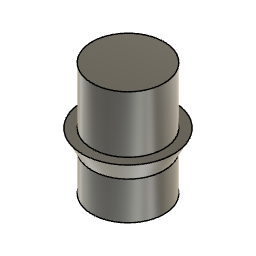
Final_CAD_Assembly (Autodesk Fusion 360 archive; units mm, degrees)
design "Button"
Autodesk Fusion 360 part; units mm, degrees
(part 1 of 3)
sketch "Sketch1" plane through (0, 0, 0) normal (0, 1, 0) x (1, 0, 0)
  line L0 (0, 0) -> (3.8, 0)
  line L1 (3.8, 0) -> (3.8, -12)
  line L2 (3.8, -12) -> (0, -12)
  line L3 (0, -12) -> (0, 0)
  line L4 (3.8, -6) -> (4.8, -6)
  line L5 (4.8, -6) -> (3.8, -4)
  line L6 (0, -0.5823) -> (0, -13.8484) construction
  dimension "d1" = 3.8
  dimension "d2" = 12
  dimension "d3" = 6
  dimension "d4" = 1
  dimension "d5" = 4
  constraint horizontal L0
  constraint vertical L1
  constraint horizontal L2
  constraint vertical L3
  constraint coincident L0.start L3.end
  constraint coincident L1 L4.start
  constraint perpendicular L1 L4
  constraint coincident L1 L5.end
  constraint coincident L3 L6.start
  constraint perpendicular L0 L6
  measures "d1" distance of L0.start L0.end
  measures "d2" distance of L0.start L2.end
  measures "d3" distance of L0 L4
  measures "d4" distance of L4.start L4.end
  measures "d5" distance of L0 L5.end
revolve "Revolve1" add sketch "Sketch1" angle 360 about axis through (0, 0, 0.5823) along (0, 0, 1)

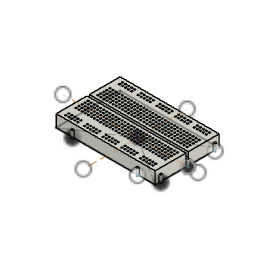
design "Breadboard"
Autodesk Fusion 360 part; units mm, degrees
sketch "Sketch1" plane through (0, 0, 0) normal (0, 0, 1) x (1, 0, 0)
  line L0 (41, 26.5) -> (-41, 26.5)
  line L1 (-41, 26.5) -> (-41, -26.5)
  line L2 (-41, -26.5) -> (41, -26.5)
  line L3 (41, -26.5) -> (41, 26.5)
  line L4 (41, 26.5) -> (-41, -26.5) construction
  line L5 (-41, 26.5) -> (41, -26.5) construction
  circle A0 centre (-27, -27.1) radius 1
  line L6 (0, 41) -> (0, -45) construction
  line L7 (50, 0) -> (-62, 0) construction
  circle A1 centre (27, -27.1) radius 1
  circle A2 centre (41.6, 0) radius 1
  circle A3 centre (41.6, -22.5) radius 1
  circle A4 centre (41.6, 22.5) radius 1
  dimension "d1" = 82
  dimension "d2" = 53
  dimension "d43" = 14
  dimension "d44" = 0.6
  dimension "d45" = 2
  dimension "d46" = 2
  dimension "d47" = 0.6
  dimension "d48" = 2
  dimension "d49" = 0.6
  dimension "d50" = 4
  constraint horizontal L0
  constraint perpendicular L0 L1
  constraint parallel L0 L2
  constraint parallel L1 L3
  constraint coincident L4 origin
  constraint coincident L5 origin
  constraint perpendicular L0 L6
  constraint perpendicular L3 L7
  constraint symmetric A0 L6 A1
  constraint coincident L7 A2.centre
  constraint symmetric L7 A3 A4
  measures "d1" distance of L0.start L0.end
  measures "d2" distance of L0.end L1.end
  measures "d43" distance of L1 A0.centre
  measures "d44" distance of L2 A0.centre
  measures "d45" diameter of A0
  measures "d46" diameter of A2
  measures "d47" distance of L3 A2.centre
  measures "d48" diameter of A3
  measures "d49" distance of L3 A3.centre
  measures "d50" distance of L2 A3.centre
extrude "Extrude1" add sketch "Sketch1" along normal blind 10 contours L0 L1 L2 L3 A0 A1 A2 A3 A4 | L3 A4 | L2 A0 | L3 A2 | L2 A1 | L3 A3 picked at (40.7957, 22.4762) picked at (-27.2307, -26.3971) picked at (40.7619, 0.2211) picked at (26.7693, -26.3971) picked at (40.7403, -22.5708)
sketch "Sketch2" plane through (0, 0, 10) normal (0, 0, 1) x (-1, 0, 0)
  line L0 (-41, 26.5) -> (-41, -26.5)
  line L1 (-41, -26.5) -> (41, -26.5)
  line L2 (41, -26.5) -> (41, 26.5)
  line L3 (41, 26.5) -> (-41, 26.5)
  line L4 (-41, -1) -> (41, -1)
  line L5 (41, -1) -> (41, 1)
  line L6 (41, 1) -> (-41, 1)
  line L7 (-41, 1) -> (-41, -1)
  line L8 (-41, -1) -> (41, 1) construction
  line L9 (41, -1) -> (-41, 1) construction
  line L10 (35.5, 23) -> (36.5, 23)
  line L11 (36.5, 23) -> (36.5, 24)
  line L12 (36.5, 24) -> (35.5, 24)
  line L13 (35.5, 24) -> (35.5, 23)
  line L14 (35.5, 23) -> (36.5, 24) construction
  line L15 (36.5, 23) -> (35.5, 24) construction
  line L16 (33, 24) -> (33, 23)
  line L17 (33, 23) -> (34, 23)
  line L18 (34, 23) -> (34, 24)
  line L19 (34, 24) -> (33, 24)
  line L20 (30.5, 24) -> (30.5, 23)
  line L21 (30.5, 23) -> (31.5, 23)
  line L22 (31.5, 23) -> (31.5, 24)
  line L23 (31.5, 24) -> (30.5, 24)
  line L24 (28, 24) -> (28, 23)
  line L25 (28, 23) -> (29, 23)
  line L26 (29, 23) -> (29, 24)
  line L27 (29, 24) -> (28, 24)
  line L28 (25.5, 24) -> (25.5, 23)
  line L29 (25.5, 23) -> (26.5, 23)
  line L30 (26.5, 23) -> (26.5, 24)
  line L31 (26.5, 24) -> (25.5, 24)
  line L32 (35.5, 21.5) -> (35.5, 20.5)
  line L33 (35.5, 20.5) -> (36.5, 20.5)
  line L34 (36.5, 20.5) -> (36.5, 21.5)
  line L35 (36.5, 21.5) -> (35.5, 21.5)
  line L36 (33, 21.5) -> (33, 20.5)
  line L37 (33, 20.5) -> (34, 20.5)
  line L38 (34, 20.5) -> (34, 21.5)
  line L39 (34, 21.5) -> (33, 21.5)
  line L40 (30.5, 21.5) -> (30.5, 20.5)
  line L41 (30.5, 20.5) -> (31.5, 20.5)
  line L42 (31.5, 20.5) -> (31.5, 21.5)
  line L43 (31.5, 21.5) -> (30.5, 21.5)
  line L44 (28, 21.5) -> (28, 20.5)
  line L45 (28, 20.5) -> (29, 20.5)
  line L46 (29, 20.5) -> (29, 21.5)
  line L47 (29, 21.5) -> (28, 21.5)
  line L48 (25.5, 21.5) -> (25.5, 20.5)
  line L49 (25.5, 20.5) -> (26.5, 20.5)
  line L50 (26.5, 20.5) -> (26.5, 21.5)
  line L51 (26.5, 21.5) -> (25.5, 21.5)
  line L52 (17.5, 23) -> (18.5, 23)
  line L53 (12.5, 24) -> (12.5, 23)
  line L54 (20, 23) -> (21, 23)
  line L55 (16, 21.5) -> (15, 21.5)
  line L56 (13.5, 23) -> (13.5, 24)
  line L57 (12.5, 21.5) -> (12.5, 20.5)
  line L58 (20, 23) -> (21, 24) construction
  line L59 (12.5, 23) -> (13.5, 23)
  line L60 (20, 20.5) -> (21, 20.5)
  line L61 (21, 24) -> (20, 24)
  line L62 (18.5, 23) -> (18.5, 24)
  line L63 (20, 24) -> (20, 23)
  line L64 (12.5, 20.5) -> (13.5, 20.5)
  line L65 (16, 23) -> (16, 24)
  line L66 (15, 23) -> (16, 23)
  line L67 (18.5, 20.5) -> (18.5, 21.5)
  line L68 (15, 21.5) -> (15, 20.5)
  line L69 (13.5, 24) -> (12.5, 24)
  line L70 (16, 24) -> (15, 24)
  line L71 (13.5, 21.5) -> (12.5, 21.5)
  line L72 (21, 21.5) -> (20, 21.5)
  line L73 (21, 20.5) -> (21, 21.5)
  line L74 (21, 23) -> (21, 24)
  line L75 (10, 21.5) -> (10, 20.5)
  line L76 (11, 23) -> (11, 24)
  line L77 (11, 24) -> (10, 24)
  line L78 (10, 24) -> (10, 23)
  line L79 (11, 21.5) -> (10, 21.5)
  line L80 (11, 20.5) -> (11, 21.5)
  line L81 (10, 23) -> (11, 23)
  line L82 (18.5, 24) -> (17.5, 24)
  line L83 (15, 20.5) -> (16, 20.5)
  line L84 (15, 24) -> (15, 23)
  line L85 (20, 21.5) -> (20, 20.5)
  line L86 (17.5, 24) -> (17.5, 23)
  line L87 (17.5, 21.5) -> (17.5, 20.5)
  line L88 (21, 23) -> (20, 24) construction
  line L89 (13.5, 20.5) -> (13.5, 21.5)
  line L90 (16, 20.5) -> (16, 21.5)
  line L91 (18.5, 21.5) -> (17.5, 21.5)
  line L92 (17.5, 20.5) -> (18.5, 20.5)
  line L93 (10, 20.5) -> (11, 20.5)
  line L94 (2, 23) -> (3, 23)
  line L95 (-3, 24) -> (-3, 23)
  line L96 (4.5, 23) -> (5.5, 23)
  line L97 (0.5, 21.5) -> (-0.5, 21.5)
  line L98 (-2, 23) -> (-2, 24)
  line L99 (-3, 21.5) -> (-3, 20.5)
  line L100 (4.5, 23) -> (5.5, 24) construction
  line L101 (-3, 23) -> (-2, 23)
  line L102 (4.5, 20.5) -> (5.5, 20.5)
  line L103 (5.5, 24) -> (4.5, 24)
  line L104 (3, 23) -> (3, 24)
  line L105 (4.5, 24) -> (4.5, 23)
  line L106 (-3, 20.5) -> (-2, 20.5)
  line L107 (0.5, 23) -> (0.5, 24)
  line L108 (-0.5, 23) -> (0.5, 23)
  line L109 (3, 20.5) -> (3, 21.5)
  line L110 (-0.5, 21.5) -> (-0.5, 20.5)
  line L111 (-2, 24) -> (-3, 24)
  line L112 (0.5, 24) -> (-0.5, 24)
  line L113 (-2, 21.5) -> (-3, 21.5)
  line L114 (5.5, 21.5) -> (4.5, 21.5)
  line L115 (5.5, 20.5) -> (5.5, 21.5)
  line L116 (5.5, 23) -> (5.5, 24)
  line L117 (-5.5, 21.5) -> (-5.5, 20.5)
  line L118 (-4.5, 23) -> (-4.5, 24)
  line L119 (-4.5, 24) -> (-5.5, 24)
  line L120 (-5.5, 24) -> (-5.5, 23)
  line L121 (-4.5, 21.5) -> (-5.5, 21.5)
  line L122 (-4.5, 20.5) -> (-4.5, 21.5)
  line L123 (-5.5, 23) -> (-4.5, 23)
  line L124 (3, 24) -> (2, 24)
  line L125 (-0.5, 20.5) -> (0.5, 20.5)
  line L126 (-0.5, 24) -> (-0.5, 23)
  line L127 (4.5, 21.5) -> (4.5, 20.5)
  line L128 (2, 24) -> (2, 23)
  line L129 (2, 21.5) -> (2, 20.5)
  line L130 (5.5, 23) -> (4.5, 24) construction
  line L131 (-2, 20.5) -> (-2, 21.5)
  line L132 (0.5, 20.5) -> (0.5, 21.5)
  line L133 (3, 21.5) -> (2, 21.5)
  line L134 (2, 20.5) -> (3, 20.5)
  line L135 (-5.5, 20.5) -> (-4.5, 20.5)
  line L136 (-13.5, 23) -> (-12.5, 23)
  line L137 (-18.5, 24) -> (-18.5, 23)
  line L138 (-11, 23) -> (-10, 23)
  line L139 (-15, 21.5) -> (-16, 21.5)
  line L140 (-17.5, 23) -> (-17.5, 24)
  line L141 (-18.5, 21.5) -> (-18.5, 20.5)
  line L142 (-11, 23) -> (-10, 24) construction
  line L143 (-18.5, 23) -> (-17.5, 23)
  line L144 (-11, 20.5) -> (-10, 20.5)
  line L145 (-10, 24) -> (-11, 24)
  line L146 (-12.5, 23) -> (-12.5, 24)
  line L147 (-11, 24) -> (-11, 23)
  line L148 (-18.5, 20.5) -> (-17.5, 20.5)
  line L149 (-15, 23) -> (-15, 24)
  line L150 (-16, 23) -> (-15, 23)
  line L151 (-12.5, 20.5) -> (-12.5, 21.5)
  line L152 (-16, 21.5) -> (-16, 20.5)
  line L153 (-17.5, 24) -> (-18.5, 24)
  line L154 (-15, 24) -> (-16, 24)
  line L155 (-17.5, 21.5) -> (-18.5, 21.5)
  line L156 (-10, 21.5) -> (-11, 21.5)
  line L157 (-10, 20.5) -> (-10, 21.5)
  line L158 (-10, 23) -> (-10, 24)
  line L159 (-21, 21.5) -> (-21, 20.5)
  line L160 (-20, 23) -> (-20, 24)
  line L161 (-20, 24) -> (-21, 24)
  line L162 (-21, 24) -> (-21, 23)
  line L163 (-20, 21.5) -> (-21, 21.5)
  line L164 (-20, 20.5) -> (-20, 21.5)
  line L165 (-21, 23) -> (-20, 23)
  line L166 (-12.5, 24) -> (-13.5, 24)
  line L167 (-16, 20.5) -> (-15, 20.5)
  line L168 (-16, 24) -> (-16, 23)
  line L169 (-11, 21.5) -> (-11, 20.5)
  line L170 (-13.5, 24) -> (-13.5, 23)
  line L171 (-13.5, 21.5) -> (-13.5, 20.5)
  line L172 (-10, 23) -> (-11, 24) construction
  line L173 (-17.5, 20.5) -> (-17.5, 21.5)
  line L174 (-15, 20.5) -> (-15, 21.5)
  line L175 (-12.5, 21.5) -> (-13.5, 21.5)
  line L176 (-13.5, 20.5) -> (-12.5, 20.5)
  line L177 (-21, 20.5) -> (-20, 20.5)
  line L178 (-29, 23) -> (-28, 23)
  line L179 (-34, 24) -> (-34, 23)
  line L180 (-26.5, 23) -> (-25.5, 23)
  line L181 (-30.5, 21.5) -> (-31.5, 21.5)
  line L182 (-33, 23) -> (-33, 24)
  line L183 (-34, 21.5) -> (-34, 20.5)
  line L184 (-26.5, 23) -> (-25.5, 24) construction
  line L185 (-34, 23) -> (-33, 23)
  line L186 (-26.5, 20.5) -> (-25.5, 20.5)
  line L187 (-25.5, 24) -> (-26.5, 24)
  line L188 (-28, 23) -> (-28, 24)
  line L189 (-26.5, 24) -> (-26.5, 23)
  line L190 (-34, 20.5) -> (-33, 20.5)
  line L191 (-30.5, 23) -> (-30.5, 24)
  line L192 (-31.5, 23) -> (-30.5, 23)
  line L193 (-28, 20.5) -> (-28, 21.5)
  line L194 (-31.5, 21.5) -> (-31.5, 20.5)
  line L195 (-33, 24) -> (-34, 24)
  line L196 (-30.5, 24) -> (-31.5, 24)
  line L197 (-33, 21.5) -> (-34, 21.5)
  line L198 (-25.5, 21.5) -> (-26.5, 21.5)
  line L199 (-25.5, 20.5) -> (-25.5, 21.5)
  line L200 (-25.5, 23) -> (-25.5, 24)
  line L201 (-36.5, 21.5) -> (-36.5, 20.5)
  line L202 (-35.5, 23) -> (-35.5, 24)
  line L203 (-35.5, 24) -> (-36.5, 24)
  line L204 (-36.5, 24) -> (-36.5, 23)
  line L205 (-35.5, 21.5) -> (-36.5, 21.5)
  line L206 (-35.5, 20.5) -> (-35.5, 21.5)
  line L207 (-36.5, 23) -> (-35.5, 23)
  line L208 (-28, 24) -> (-29, 24)
  line L209 (-31.5, 20.5) -> (-30.5, 20.5)
  line L210 (-31.5, 24) -> (-31.5, 23)
  line L211 (-26.5, 21.5) -> (-26.5, 20.5)
  line L212 (-29, 24) -> (-29, 23)
  line L213 (-29, 21.5) -> (-29, 20.5)
  line L214 (-25.5, 23) -> (-26.5, 24) construction
  line L215 (-33, 20.5) -> (-33, 21.5)
  line L216 (-30.5, 20.5) -> (-30.5, 21.5)
  line L217 (-28, 21.5) -> (-29, 21.5)
  line L218 (-29, 20.5) -> (-28, 20.5)
  line L219 (-36.5, 20.5) -> (-35.5, 20.5)
  line L220 (36.5, 4.5) -> (37.5, 4.5)
  line L221 (37.5, 4.5) -> (37.5, 3.5)
  line L222 (37.5, 3.5) -> (36.5, 3.5)
  line L223 (36.5, 3.5) -> (36.5, 4.5)
  line L224 (36.5, 4.5) -> (37.5, 3.5) construction
  line L225 (37.5, 4.5) -> (36.5, 3.5) construction
  line L226 (33.9483, 3.5) -> (33.9483, 4.5)
  line L227 (34.9483, 3.5) -> (33.9483, 3.5)
  line L228 (34.9483, 4.5) -> (34.9483, 3.5)
  line L229 (33.9483, 4.5) -> (34.9483, 4.5)
  line L230 (31.3966, 3.5) -> (31.3966, 4.5)
  line L231 (32.3966, 3.5) -> (31.3966, 3.5)
  line L232 (32.3966, 4.5) -> (32.3966, 3.5)
  line L233 (31.3966, 4.5) -> (32.3966, 4.5)
  line L234 (28.8448, 3.5) -> (28.8448, 4.5)
  line L235 (29.8448, 3.5) -> (28.8448, 3.5)
  line L236 (29.8448, 4.5) -> (29.8448, 3.5)
  line L237 (28.8448, 4.5) -> (29.8448, 4.5)
  line L238 (26.2931, 3.5) -> (26.2931, 4.5)
  line L239 (27.2931, 3.5) -> (26.2931, 3.5)
  line L240 (27.2931, 4.5) -> (27.2931, 3.5)
  line L241 (26.2931, 4.5) -> (27.2931, 4.5)
  line L242 (23.7414, 3.5) -> (23.7414, 4.5)
  line L243 (24.7414, 3.5) -> (23.7414, 3.5)
  line L244 (24.7414, 4.5) -> (24.7414, 3.5)
  line L245 (23.7414, 4.5) -> (24.7414, 4.5)
  line L246 (21.1897, 3.5) -> (21.1897, 4.5)
  line L247 (22.1897, 3.5) -> (21.1897, 3.5)
  line L248 (22.1897, 4.5) -> (22.1897, 3.5)
  line L249 (21.1897, 4.5) -> (22.1897, 4.5)
  line L250 (18.6379, 3.5) -> (18.6379, 4.5)
  line L251 (19.6379, 3.5) -> (18.6379, 3.5)
  line L252 (19.6379, 4.5) -> (19.6379, 3.5)
  line L253 (18.6379, 4.5) -> (19.6379, 4.5)
  line L254 (16.0862, 3.5) -> (16.0862, 4.5)
  line L255 (17.0862, 3.5) -> (16.0862, 3.5)
  line L256 (17.0862, 4.5) -> (17.0862, 3.5)
  line L257 (16.0862, 4.5) -> (17.0862, 4.5)
  line L258 (13.5345, 3.5) -> (13.5345, 4.5)
  line L259 (14.5345, 3.5) -> (13.5345, 3.5)
  line L260 (14.5345, 4.5) -> (14.5345, 3.5)
  line L261 (13.5345, 4.5) -> (14.5345, 4.5)
  line L262 (10.9828, 3.5) -> (10.9828, 4.5)
  line L263 (11.9828, 3.5) -> (10.9828, 3.5)
  line L264 (11.9828, 4.5) -> (11.9828, 3.5)
  line L265 (10.9828, 4.5) -> (11.9828, 4.5)
  line L266 (8.431, 3.5) -> (8.431, 4.5)
  line L267 (9.431, 3.5) -> (8.431, 3.5)
  line L268 (9.431, 4.5) -> (9.431, 3.5)
  line L269 (8.431, 4.5) -> (9.431, 4.5)
  line L270 (5.8793, 3.5) -> (5.8793, 4.5)
  line L271 (6.8793, 3.5) -> (5.8793, 3.5)
  line L272 (6.8793, 4.5) -> (6.8793, 3.5)
  line L273 (5.8793, 4.5) -> (6.8793, 4.5)
  line L274 (3.3276, 3.5) -> (3.3276, 4.5)
  line L275 (4.3276, 3.5) -> (3.3276, 3.5)
  line L276 (4.3276, 4.5) -> (4.3276, 3.5)
  line L277 (3.3276, 4.5) -> (4.3276, 4.5)
  line L278 (0.7759, 3.5) -> (0.7759, 4.5)
  line L279 (1.7759, 3.5) -> (0.7759, 3.5)
  line L280 (1.7759, 4.5) -> (1.7759, 3.5)
  line L281 (0.7759, 4.5) -> (1.7759, 4.5)
  line L282 (-1.7759, 3.5) -> (-1.7759, 4.5)
  line L283 (-0.7759, 3.5) -> (-1.7759, 3.5)
  line L284 (-0.7759, 4.5) -> (-0.7759, 3.5)
  line L285 (-1.7759, 4.5) -> (-0.7759, 4.5)
  line L286 (-4.3276, 3.5) -> (-4.3276, 4.5)
  line L287 (-3.3276, 3.5) -> (-4.3276, 3.5)
  line L288 (-3.3276, 4.5) -> (-3.3276, 3.5)
  line L289 (-4.3276, 4.5) -> (-3.3276, 4.5)
  line L290 (-6.8793, 3.5) -> (-6.8793, 4.5)
  line L291 (-5.8793, 3.5) -> (-6.8793, 3.5)
  line L292 (-5.8793, 4.5) -> (-5.8793, 3.5)
  line L293 (-6.8793, 4.5) -> (-5.8793, 4.5)
  line L294 (-9.431, 3.5) -> (-9.431, 4.5)
  line L295 (-8.431, 3.5) -> (-9.431, 3.5)
  line L296 (-8.431, 4.5) -> (-8.431, 3.5)
  line L297 (-9.431, 4.5) -> (-8.431, 4.5)
  line L298 (-11.9828, 3.5) -> (-11.9828, 4.5)
  line L299 (-10.9828, 3.5) -> (-11.9828, 3.5)
  line L300 (-10.9828, 4.5) -> (-10.9828, 3.5)
  line L301 (-11.9828, 4.5) -> (-10.9828, 4.5)
  line L302 (-14.5345, 3.5) -> (-14.5345, 4.5)
  line L303 (-13.5345, 3.5) -> (-14.5345, 3.5)
  line L304 (-13.5345, 4.5) -> (-13.5345, 3.5)
  line L305 (-14.5345, 4.5) -> (-13.5345, 4.5)
  line L306 (-17.0862, 3.5) -> (-17.0862, 4.5)
  line L307 (-16.0862, 3.5) -> (-17.0862, 3.5)
  line L308 (-16.0862, 4.5) -> (-16.0862, 3.5)
  line L309 (-17.0862, 4.5) -> (-16.0862, 4.5)
  line L310 (-19.6379, 3.5) -> (-19.6379, 4.5)
  line L311 (-18.6379, 3.5) -> (-19.6379, 3.5)
  line L312 (-18.6379, 4.5) -> (-18.6379, 3.5)
  line L313 (-19.6379, 4.5) -> (-18.6379, 4.5)
  line L314 (-22.1897, 3.5) -> (-22.1897, 4.5)
  line L315 (-21.1897, 3.5) -> (-22.1897, 3.5)
  line L316 (-21.1897, 4.5) -> (-21.1897, 3.5)
  line L317 (-22.1897, 4.5) -> (-21.1897, 4.5)
  line L318 (-24.7414, 3.5) -> (-24.7414, 4.5)
  line L319 (-23.7414, 3.5) -> (-24.7414, 3.5)
  line L320 (-23.7414, 4.5) -> (-23.7414, 3.5)
  line L321 (-24.7414, 4.5) -> (-23.7414, 4.5)
  line L322 (-27.2931, 3.5) -> (-27.2931, 4.5)
  line L323 (-26.2931, 3.5) -> (-27.2931, 3.5)
  line L324 (-26.2931, 4.5) -> (-26.2931, 3.5)
  line L325 (-27.2931, 4.5) -> (-26.2931, 4.5)
  line L326 (-29.8448, 3.5) -> (-29.8448, 4.5)
  line L327 (-28.8448, 3.5) -> (-29.8448, 3.5)
  line L328 (-28.8448, 4.5) -> (-28.8448, 3.5)
  line L329 (-29.8448, 4.5) -> (-28.8448, 4.5)
  line L330 (-32.3966, 3.5) -> (-32.3966, 4.5)
  line L331 (-31.3966, 3.5) -> (-32.3966, 3.5)
  line L332 (-31.3966, 4.5) -> (-31.3966, 3.5)
  line L333 (-32.3966, 4.5) -> (-31.3966, 4.5)
  line L334 (-34.9483, 3.5) -> (-34.9483, 4.5)
  line L335 (-33.9483, 3.5) -> (-34.9483, 3.5)
  line L336 (-33.9483, 4.5) -> (-33.9483, 3.5)
  line L337 (-34.9483, 4.5) -> (-33.9483, 4.5)
  line L338 (-37.5, 3.5) -> (-37.5, 4.5)
  line L339 (-36.5, 3.5) -> (-37.5, 3.5)
  line L340 (-36.5, 4.5) -> (-36.5, 3.5)
  line L341 (-37.5, 4.5) -> (-36.5, 4.5)
  line L342 (36.5, 6) -> (36.5, 7)
  line L343 (37.5, 6) -> (36.5, 6)
  line L344 (37.5, 7) -> (37.5, 6)
  line L345 (36.5, 7) -> (37.5, 7)
  line L346 (33.9483, 6) -> (33.9483, 7)
  line L347 (34.9483, 6) -> (33.9483, 6)
  line L348 (34.9483, 7) -> (34.9483, 6)
  line L349 (33.9483, 7) -> (34.9483, 7)
  line L350 (31.3966, 6) -> (31.3966, 7)
  line L351 (32.3966, 6) -> (31.3966, 6)
  line L352 (32.3966, 7) -> (32.3966, 6)
  line L353 (31.3966, 7) -> (32.3966, 7)
  line L354 (28.8448, 6) -> (28.8448, 7)
  line L355 (29.8448, 6) -> (28.8448, 6)
  line L356 (29.8448, 7) -> (29.8448, 6)
  line L357 (28.8448, 7) -> (29.8448, 7)
  line L358 (26.2931, 6) -> (26.2931, 7)
  line L359 (27.2931, 6) -> (26.2931, 6)
  line L360 (27.2931, 7) -> (27.2931, 6)
  line L361 (26.2931, 7) -> (27.2931, 7)
  line L362 (23.7414, 6) -> (23.7414, 7)
  line L363 (24.7414, 6) -> (23.7414, 6)
  line L364 (24.7414, 7) -> (24.7414, 6)
  line L365 (23.7414, 7) -> (24.7414, 7)
  line L366 (21.1897, 6) -> (21.1897, 7)
  line L367 (22.1897, 6) -> (21.1897, 6)
  line L368 (22.1897, 7) -> (22.1897, 6)
  line L369 (21.1897, 7) -> (22.1897, 7)
  line L370 (18.6379, 6) -> (18.6379, 7)
  line L371 (19.6379, 6) -> (18.6379, 6)
  line L372 (19.6379, 7) -> (19.6379, 6)
  line L373 (18.6379, 7) -> (19.6379, 7)
  line L374 (16.0862, 6) -> (16.0862, 7)
  line L375 (17.0862, 6) -> (16.0862, 6)
  line L376 (17.0862, 7) -> (17.0862, 6)
  line L377 (16.0862, 7) -> (17.0862, 7)
  line L378 (13.5345, 6) -> (13.5345, 7)
  line L379 (14.5345, 6) -> (13.5345, 6)
  line L380 (14.5345, 7) -> (14.5345, 6)
  line L381 (13.5345, 7) -> (14.5345, 7)
  line L382 (10.9828, 6) -> (10.9828, 7)
  line L383 (11.9828, 6) -> (10.9828, 6)
  line L384 (11.9828, 7) -> (11.9828, 6)
  line L385 (10.9828, 7) -> (11.9828, 7)
  line L386 (8.431, 6) -> (8.431, 7)
  line L387 (9.431, 6) -> (8.431, 6)
  line L388 (9.431, 7) -> (9.431, 6)
  line L389 (8.431, 7) -> (9.431, 7)
  line L390 (5.8793, 6) -> (5.8793, 7)
  line L391 (6.8793, 6) -> (5.8793, 6)
  line L392 (6.8793, 7) -> (6.8793, 6)
  line L393 (5.8793, 7) -> (6.8793, 7)
  line L394 (3.3276, 6) -> (3.3276, 7)
  line L395 (4.3276, 6) -> (3.3276, 6)
  line L396 (4.3276, 7) -> (4.3276, 6)
  line L397 (3.3276, 7) -> (4.3276, 7)
  line L398 (0.7759, 6) -> (0.7759, 7)
  line L399 (1.7759, 6) -> (0.7759, 6)
  line L400 (1.7759, 7) -> (1.7759, 6)
  line L401 (0.7759, 7) -> (1.7759, 7)
  line L402 (-1.7759, 6) -> (-1.7759, 7)
  line L403 (-0.7759, 6) -> (-1.7759, 6)
  line L404 (-0.7759, 7) -> (-0.7759, 6)
  line L405 (-1.7759, 7) -> (-0.7759, 7)
  line L406 (-4.3276, 6) -> (-4.3276, 7)
  line L407 (-3.3276, 6) -> (-4.3276, 6)
  line L408 (-3.3276, 7) -> (-3.3276, 6)
  line L409 (-4.3276, 7) -> (-3.3276, 7)
  line L410 (-6.8793, 6) -> (-6.8793, 7)
  line L411 (-5.8793, 6) -> (-6.8793, 6)
  line L412 (-5.8793, 7) -> (-5.8793, 6)
  line L413 (-6.8793, 7) -> (-5.8793, 7)
  line L414 (-9.431, 6) -> (-9.431, 7)
  line L415 (-8.431, 6) -> (-9.431, 6)
  line L416 (-8.431, 7) -> (-8.431, 6)
  line L417 (-9.431, 7) -> (-8.431, 7)
  line L418 (-11.9828, 6) -> (-11.9828, 7)
  line L419 (-10.9828, 6) -> (-11.9828, 6)
  line L420 (-10.9828, 7) -> (-10.9828, 6)
  line L421 (-11.9828, 7) -> (-10.9828, 7)
  line L422 (-14.5345, 6) -> (-14.5345, 7)
  line L423 (-13.5345, 6) -> (-14.5345, 6)
  line L424 (-13.5345, 7) -> (-13.5345, 6)
  line L425 (-14.5345, 7) -> (-13.5345, 7)
  line L426 (-17.0862, 6) -> (-17.0862, 7)
  line L427 (-16.0862, 6) -> (-17.0862, 6)
  line L428 (-16.0862, 7) -> (-16.0862, 6)
  line L429 (-17.0862, 7) -> (-16.0862, 7)
  line L430 (-19.6379, 6) -> (-19.6379, 7)
  line L431 (-18.6379, 6) -> (-19.6379, 6)
  line L432 (-18.6379, 7) -> (-18.6379, 6)
  line L433 (-19.6379, 7) -> (-18.6379, 7)
  line L434 (-22.1897, 6) -> (-22.1897, 7)
  line L435 (-21.1897, 6) -> (-22.1897, 6)
  line L436 (-21.1897, 7) -> (-21.1897, 6)
  line L437 (-22.1897, 7) -> (-21.1897, 7)
  line L438 (-24.7414, 6) -> (-24.7414, 7)
  line L439 (-23.7414, 6) -> (-24.7414, 6)
  line L440 (-23.7414, 7) -> (-23.7414, 6)
  line L441 (-24.7414, 7) -> (-23.7414, 7)
  line L442 (-27.2931, 6) -> (-27.2931, 7)
  line L443 (-26.2931, 6) -> (-27.2931, 6)
  line L444 (-26.2931, 7) -> (-26.2931, 6)
  line L445 (-27.2931, 7) -> (-26.2931, 7)
  line L446 (-29.8448, 6) -> (-29.8448, 7)
  line L447 (-28.8448, 6) -> (-29.8448, 6)
  line L448 (-28.8448, 7) -> (-28.8448, 6)
  line L449 (-29.8448, 7) -> (-28.8448, 7)
  line L450 (-32.3966, 6) -> (-32.3966, 7)
  line L451 (-31.3966, 6) -> (-32.3966, 6)
  line L452 (-31.3966, 7) -> (-31.3966, 6)
  line L453 (-32.3966, 7) -> (-31.3966, 7)
  line L454 (-34.9483, 6) -> (-34.9483, 7)
  line L455 (-33.9483, 6) -> (-34.9483, 6)
  line L456 (-33.9483, 7) -> (-33.9483, 6)
  line L457 (-34.9483, 7) -> (-33.9483, 7)
  line L458 (-37.5, 6) -> (-37.5, 7)
  line L459 (-36.5, 6) -> (-37.5, 6)
  line L460 (-36.5, 7) -> (-36.5, 6)
  line L461 (-37.5, 7) -> (-36.5, 7)
  line L462 (36.5, 8.5) -> (36.5, 9.5)
  line L463 (37.5, 8.5) -> (36.5, 8.5)
  line L464 (37.5, 9.5) -> (37.5, 8.5)
  line L465 (36.5, 9.5) -> (37.5, 9.5)
  line L466 (33.9483, 8.5) -> (33.9483, 9.5)
  line L467 (34.9483, 8.5) -> (33.9483, 8.5)
  line L468 (34.9483, 9.5) -> (34.9483, 8.5)
  line L469 (33.9483, 9.5) -> (34.9483, 9.5)
  line L470 (31.3966, 8.5) -> (31.3966, 9.5)
  line L471 (32.3966, 8.5) -> (31.3966, 8.5)
  line L472 (32.3966, 9.5) -> (32.3966, 8.5)
  line L473 (31.3966, 9.5) -> (32.3966, 9.5)
  line L474 (28.8448, 8.5) -> (28.8448, 9.5)
  line L475 (29.8448, 8.5) -> (28.8448, 8.5)
  line L476 (29.8448, 9.5) -> (29.8448, 8.5)
  line L477 (28.8448, 9.5) -> (29.8448, 9.5)
  line L478 (26.2931, 8.5) -> (26.2931, 9.5)
  line L479 (27.2931, 8.5) -> (26.2931, 8.5)
  line L480 (27.2931, 9.5) -> (27.2931, 8.5)
  line L481 (26.2931, 9.5) -> (27.2931, 9.5)
  line L482 (23.7414, 8.5) -> (23.7414, 9.5)
  line L483 (24.7414, 8.5) -> (23.7414, 8.5)
  line L484 (24.7414, 9.5) -> (24.7414, 8.5)
  line L485 (23.7414, 9.5) -> (24.7414, 9.5)
  line L486 (21.1897, 8.5) -> (21.1897, 9.5)
  line L487 (22.1897, 8.5) -> (21.1897, 8.5)
  line L488 (22.1897, 9.5) -> (22.1897, 8.5)
  line L489 (21.1897, 9.5) -> (22.1897, 9.5)
  line L490 (18.6379, 8.5) -> (18.6379, 9.5)
  line L491 (19.6379, 8.5) -> (18.6379, 8.5)
  line L492 (19.6379, 9.5) -> (19.6379, 8.5)
  line L493 (18.6379, 9.5) -> (19.6379, 9.5)
  line L494 (16.0862, 8.5) -> (16.0862, 9.5)
  line L495 (17.0862, 8.5) -> (16.0862, 8.5)
  line L496 (17.0862, 9.5) -> (17.0862, 8.5)
  line L497 (16.0862, 9.5) -> (17.0862, 9.5)
  line L498 (13.5345, 8.5) -> (13.5345, 9.5)
  line L499 (14.5345, 8.5) -> (13.5345, 8.5)
  line L500 (14.5345, 9.5) -> (14.5345, 8.5)
  line L501 (13.5345, 9.5) -> (14.5345, 9.5)
  line L502 (10.9828, 8.5) -> (10.9828, 9.5)
  line L503 (11.9828, 8.5) -> (10.9828, 8.5)
  line L504 (11.9828, 9.5) -> (11.9828, 8.5)
  line L505 (10.9828, 9.5) -> (11.9828, 9.5)
  line L506 (8.431, 8.5) -> (8.431, 9.5)
  line L507 (9.431, 8.5) -> (8.431, 8.5)
  line L508 (9.431, 9.5) -> (9.431, 8.5)
  line L509 (8.431, 9.5) -> (9.431, 9.5)
  line L510 (5.8793, 8.5) -> (5.8793, 9.5)
  line L511 (6.8793, 8.5) -> (5.8793, 8.5)
  line L512 (6.8793, 9.5) -> (6.8793, 8.5)
  line L513 (5.8793, 9.5) -> (6.8793, 9.5)
  line L514 (3.3276, 8.5) -> (3.3276, 9.5)
  line L515 (4.3276, 8.5) -> (3.3276, 8.5)
  line L516 (4.3276, 9.5) -> (4.3276, 8.5)
  line L517 (3.3276, 9.5) -> (4.3276, 9.5)
  line L518 (0.7759, 8.5) -> (0.7759, 9.5)
  line L519 (1.7759, 8.5) -> (0.7759, 8.5)
  line L520 (1.7759, 9.5) -> (1.7759, 8.5)
  line L521 (0.7759, 9.5) -> (1.7759, 9.5)
  line L522 (-1.7759, 8.5) -> (-1.7759, 9.5)
  line L523 (-0.7759, 8.5) -> (-1.7759, 8.5)
  line L524 (-0.7759, 9.5) -> (-0.7759, 8.5)
  line L525 (-1.7759, 9.5) -> (-0.7759, 9.5)
  line L526 (-4.3276, 8.5) -> (-4.3276, 9.5)
  line L527 (-3.3276, 8.5) -> (-4.3276, 8.5)
  line L528 (-3.3276, 9.5) -> (-3.3276, 8.5)
  line L529 (-4.3276, 9.5) -> (-3.3276, 9.5)
  line L530 (-6.8793, 8.5) -> (-6.8793, 9.5)
  line L531 (-5.8793, 8.5) -> (-6.8793, 8.5)
  line L532 (-5.8793, 9.5) -> (-5.8793, 8.5)
  line L533 (-6.8793, 9.5) -> (-5.8793, 9.5)
  line L534 (-9.431, 8.5) -> (-9.431, 9.5)
  line L535 (-8.431, 8.5) -> (-9.431, 8.5)
  line L536 (-8.431, 9.5) -> (-8.431, 8.5)
  line L537 (-9.431, 9.5) -> (-8.431, 9.5)
  line L538 (-11.9828, 8.5) -> (-11.9828, 9.5)
  line L539 (-10.9828, 8.5) -> (-11.9828, 8.5)
  line L540 (-10.9828, 9.5) -> (-10.9828, 8.5)
  line L541 (-11.9828, 9.5) -> (-10.9828, 9.5)
  line L542 (-14.5345, 8.5) -> (-14.5345, 9.5)
  line L543 (-13.5345, 8.5) -> (-14.5345, 8.5)
  line L544 (-13.5345, 9.5) -> (-13.5345, 8.5)
  line L545 (-14.5345, 9.5) -> (-13.5345, 9.5)
  line L546 (-17.0862, 8.5) -> (-17.0862, 9.5)
  line L547 (-16.0862, 8.5) -> (-17.0862, 8.5)
  line L548 (-16.0862, 9.5) -> (-16.0862, 8.5)
  line L549 (-17.0862, 9.5) -> (-16.0862, 9.5)
  line L550 (-19.6379, 8.5) -> (-19.6379, 9.5)
  line L551 (-18.6379, 8.5) -> (-19.6379, 8.5)
  line L552 (-18.6379, 9.5) -> (-18.6379, 8.5)
  line L553 (-19.6379, 9.5) -> (-18.6379, 9.5)
  line L554 (-22.1897, 8.5) -> (-22.1897, 9.5)
  line L555 (-21.1897, 8.5) -> (-22.1897, 8.5)
  line L556 (-21.1897, 9.5) -> (-21.1897, 8.5)
  line L557 (-22.1897, 9.5) -> (-21.1897, 9.5)
  line L558 (-24.7414, 8.5) -> (-24.7414, 9.5)
  line L559 (-23.7414, 8.5) -> (-24.7414, 8.5)
  line L560 (-23.7414, 9.5) -> (-23.7414, 8.5)
  line L561 (-24.7414, 9.5) -> (-23.7414, 9.5)
  line L562 (-27.2931, 8.5) -> (-27.2931, 9.5)
  line L563 (-26.2931, 8.5) -> (-27.2931, 8.5)
  line L564 (-26.2931, 9.5) -> (-26.2931, 8.5)
  line L565 (-27.2931, 9.5) -> (-26.2931, 9.5)
  line L566 (-29.8448, 8.5) -> (-29.8448, 9.5)
  line L567 (-28.8448, 8.5) -> (-29.8448, 8.5)
  line L568 (-28.8448, 9.5) -> (-28.8448, 8.5)
  line L569 (-29.8448, 9.5) -> (-28.8448, 9.5)
  line L570 (-32.3966, 8.5) -> (-32.3966, 9.5)
  line L571 (-31.3966, 8.5) -> (-32.3966, 8.5)
  line L572 (-31.3966, 9.5) -> (-31.3966, 8.5)
  line L573 (-32.3966, 9.5) -> (-31.3966, 9.5)
  line L574 (-34.9483, 8.5) -> (-34.9483, 9.5)
  line L575 (-33.9483, 8.5) -> (-34.9483, 8.5)
  line L576 (-33.9483, 9.5) -> (-33.9483, 8.5)
  line L577 (-34.9483, 9.5) -> (-33.9483, 9.5)
  line L578 (-37.5, 8.5) -> (-37.5, 9.5)
  line L579 (-36.5, 8.5) -> (-37.5, 8.5)
  line L580 (-36.5, 9.5) -> (-36.5, 8.5)
  line L581 (-37.5, 9.5) -> (-36.5, 9.5)
  line L582 (36.5, 11) -> (36.5, 12)
  line L583 (37.5, 11) -> (36.5, 11)
  line L584 (37.5, 12) -> (37.5, 11)
  line L585 (36.5, 12) -> (37.5, 12)
  line L586 (33.9483, 11) -> (33.9483, 12)
  line L587 (34.9483, 11) -> (33.9483, 11)
  line L588 (34.9483, 12) -> (34.9483, 11)
  line L589 (33.9483, 12) -> (34.9483, 12)
  line L590 (31.3966, 11) -> (31.3966, 12)
  line L591 (32.3966, 11) -> (31.3966, 11)
  line L592 (32.3966, 12) -> (32.3966, 11)
  line L593 (31.3966, 12) -> (32.3966, 12)
  line L594 (28.8448, 11) -> (28.8448, 12)
  line L595 (29.8448, 11) -> (28.8448, 11)
  line L596 (29.8448, 12) -> (29.8448, 11)
  line L597 (28.8448, 12) -> (29.8448, 12)
  line L598 (26.2931, 11) -> (26.2931, 12)
  line L599 (27.2931, 11) -> (26.2931, 11)
  line L600 (27.2931, 12) -> (27.2931, 11)
  line L601 (26.2931, 12) -> (27.2931, 12)
  line L602 (23.7414, 11) -> (23.7414, 12)
  line L603 (24.7414, 11) -> (23.7414, 11)
  line L604 (24.7414, 12) -> (24.7414, 11)
  line L605 (23.7414, 12) -> (24.7414, 12)
  line L606 (21.1897, 11) -> (21.1897, 12)
  line L607 (22.1897, 11) -> (21.1897, 11)
  line L608 (22.1897, 12) -> (22.1897, 11)
  line L609 (21.1897, 12) -> (22.1897, 12)
  line L610 (18.6379, 11) -> (18.6379, 12)
  line L611 (19.6379, 11) -> (18.6379, 11)
  line L612 (19.6379, 12) -> (19.6379, 11)
  line L613 (18.6379, 12) -> (19.6379, 12)
  line L614 (16.0862, 11) -> (16.0862, 12)
  line L615 (17.0862, 11) -> (16.0862, 11)
  line L616 (17.0862, 12) -> (17.0862, 11)
  line L617 (16.0862, 12) -> (17.0862, 12)
  line L618 (13.5345, 11) -> (13.5345, 12)
  line L619 (14.5345, 11) -> (13.5345, 11)
  line L620 (14.5345, 12) -> (14.5345, 11)
  line L621 (13.5345, 12) -> (14.5345, 12)
  line L622 (10.9828, 11) -> (10.9828, 12)
  line L623 (11.9828, 11) -> (10.9828, 11)
  line L624 (11.9828, 12) -> (11.9828, 11)
  line L625 (10.9828, 12) -> (11.9828, 12)
  line L626 (8.431, 11) -> (8.431, 12)
  line L627 (9.431, 11) -> (8.431, 11)
  line L628 (9.431, 12) -> (9.431, 11)
  line L629 (8.431, 12) -> (9.431, 12)
  line L630 (5.8793, 11) -> (5.8793, 12)
  line L631 (6.8793, 11) -> (5.8793, 11)
  line L632 (6.8793, 12) -> (6.8793, 11)
  line L633 (5.8793, 12) -> (6.8793, 12)
  line L634 (3.3276, 11) -> (3.3276, 12)
  line L635 (4.3276, 11) -> (3.3276, 11)
  line L636 (4.3276, 12) -> (4.3276, 11)
  line L637 (3.3276, 12) -> (4.3276, 12)
  line L638 (0.7759, 11) -> (0.7759, 12)
  line L639 (1.7759, 11) -> (0.7759, 11)
  line L640 (1.7759, 12) -> (1.7759, 11)
  line L641 (0.7759, 12) -> (1.7759, 12)
  line L642 (-1.7759, 11) -> (-1.7759, 12)
  line L643 (-0.7759, 11) -> (-1.7759, 11)
  line L644 (-0.7759, 12) -> (-0.7759, 11)
  line L645 (-1.7759, 12) -> (-0.7759, 12)
  line L646 (-4.3276, 11) -> (-4.3276, 12)
  line L647 (-3.3276, 11) -> (-4.3276, 11)
  line L648 (-3.3276, 12) -> (-3.3276, 11)
  line L649 (-4.3276, 12) -> (-3.3276, 12)
  line L650 (-6.8793, 11) -> (-6.8793, 12)
  line L651 (-5.8793, 11) -> (-6.8793, 11)
  line L652 (-5.8793, 12) -> (-5.8793, 11)
  line L653 (-6.8793, 12) -> (-5.8793, 12)
  line L654 (-9.431, 11) -> (-9.431, 12)
  line L655 (-8.431, 11) -> (-9.431, 11)
  line L656 (-8.431, 12) -> (-8.431, 11)
  line L657 (-9.431, 12) -> (-8.431, 12)
  line L658 (-11.9828, 11) -> (-11.9828, 12)
  line L659 (-10.9828, 11) -> (-11.9828, 11)
  line L660 (-10.9828, 12) -> (-10.9828, 11)
  line L661 (-11.9828, 12) -> (-10.9828, 12)
  line L662 (-14.5345, 11) -> (-14.5345, 12)
  line L663 (-13.5345, 11) -> (-14.5345, 11)
  line L664 (-13.5345, 12) -> (-13.5345, 11)
  line L665 (-14.5345, 12) -> (-13.5345, 12)
  line L666 (-17.0862, 11) -> (-17.0862, 12)
  line L667 (-16.0862, 11) -> (-17.0862, 11)
  line L668 (-16.0862, 12) -> (-16.0862, 11)
  line L669 (-17.0862, 12) -> (-16.0862, 12)
  line L670 (-19.6379, 11) -> (-19.6379, 12)
  line L671 (-18.6379, 11) -> (-19.6379, 11)
  line L672 (-18.6379, 12) -> (-18.6379, 11)
  line L673 (-19.6379, 12) -> (-18.6379, 12)
  line L674 (-22.1897, 11) -> (-22.1897, 12)
  line L675 (-21.1897, 11) -> (-22.1897, 11)
  line L676 (-21.1897, 12) -> (-21.1897, 11)
  line L677 (-22.1897, 12) -> (-21.1897, 12)
  line L678 (-24.7414, 11) -> (-24.7414, 12)
  line L679 (-23.7414, 11) -> (-24.7414, 11)
  line L680 (-23.7414, 12) -> (-23.7414, 11)
  line L681 (-24.7414, 12) -> (-23.7414, 12)
  line L682 (-27.2931, 11) -> (-27.2931, 12)
  line L683 (-26.2931, 11) -> (-27.2931, 11)
  line L684 (-26.2931, 12) -> (-26.2931, 11)
  line L685 (-27.2931, 12) -> (-26.2931, 12)
  line L686 (-29.8448, 11) -> (-29.8448, 12)
  line L687 (-28.8448, 11) -> (-29.8448, 11)
  line L688 (-28.8448, 12) -> (-28.8448, 11)
  line L689 (-29.8448, 12) -> (-28.8448, 12)
  line L690 (-32.3966, 11) -> (-32.3966, 12)
  line L691 (-31.3966, 11) -> (-32.3966, 11)
  line L692 (-31.3966, 12) -> (-31.3966, 11)
  line L693 (-32.3966, 12) -> (-31.3966, 12)
  line L694 (-34.9483, 11) -> (-34.9483, 12)
  line L695 (-33.9483, 11) -> (-34.9483, 11)
  line L696 (-33.9483, 12) -> (-33.9483, 11)
  line L697 (-34.9483, 12) -> (-33.9483, 12)
  line L698 (-37.5, 11) -> (-37.5, 12)
  line L699 (-36.5, 11) -> (-37.5, 11)
  line L700 (-36.5, 12) -> (-36.5, 11)
  line L701 (-37.5, 12) -> (-36.5, 12)
  line L702 (36.5, 13.5) -> (36.5, 14.5)
  line L703 (37.5, 13.5) -> (36.5, 13.5)
  line L704 (37.5, 14.5) -> (37.5, 13.5)
  line L705 (36.5, 14.5) -> (37.5, 14.5)
  line L706 (33.9483, 13.5) -> (33.9483, 14.5)
  line L707 (34.9483, 13.5) -> (33.9483, 13.5)
  line L708 (34.9483, 14.5) -> (34.9483, 13.5)
  line L709 (33.9483, 14.5) -> (34.9483, 14.5)
  line L710 (31.3966, 13.5) -> (31.3966, 14.5)
  line L711 (32.3966, 13.5) -> (31.3966, 13.5)
  line L712 (32.3966, 14.5) -> (32.3966, 13.5)
  line L713 (31.3966, 14.5) -> (32.3966, 14.5)
  line L714 (28.8448, 13.5) -> (28.8448, 14.5)
  line L715 (29.8448, 13.5) -> (28.8448, 13.5)
  line L716 (29.8448, 14.5) -> (29.8448, 13.5)
  line L717 (28.8448, 14.5) -> (29.8448, 14.5)
  line L718 (26.2931, 13.5) -> (26.2931, 14.5)
  line L719 (27.2931, 13.5) -> (26.2931, 13.5)
  line L720 (27.2931, 14.5) -> (27.2931, 13.5)
  line L721 (26.2931, 14.5) -> (27.2931, 14.5)
  line L722 (23.7414, 13.5) -> (23.7414, 14.5)
  line L723 (24.7414, 13.5) -> (23.7414, 13.5)
  line L724 (24.7414, 14.5) -> (24.7414, 13.5)
  line L725 (23.7414, 14.5) -> (24.7414, 14.5)
  line L726 (21.1897, 13.5) -> (21.1897, 14.5)
  line L727 (22.1897, 13.5) -> (21.1897, 13.5)
  line L728 (22.1897, 14.5) -> (22.1897, 13.5)
  line L729 (21.1897, 14.5) -> (22.1897, 14.5)
  line L730 (18.6379, 13.5) -> (18.6379, 14.5)
  line L731 (19.6379, 13.5) -> (18.6379, 13.5)
  line L732 (19.6379, 14.5) -> (19.6379, 13.5)
  line L733 (18.6379, 14.5) -> (19.6379, 14.5)
  line L734 (16.0862, 13.5) -> (16.0862, 14.5)
  line L735 (17.0862, 13.5) -> (16.0862, 13.5)
  line L736 (17.0862, 14.5) -> (17.0862, 13.5)
  line L737 (16.0862, 14.5) -> (17.0862, 14.5)
  line L738 (13.5345, 13.5) -> (13.5345, 14.5)
  line L739 (14.5345, 13.5) -> (13.5345, 13.5)
  line L740 (14.5345, 14.5) -> (14.5345, 13.5)
  line L741 (13.5345, 14.5) -> (14.5345, 14.5)
  line L742 (10.9828, 13.5) -> (10.9828, 14.5)
  line L743 (11.9828, 13.5) -> (10.9828, 13.5)
  line L744 (11.9828, 14.5) -> (11.9828, 13.5)
  line L745 (10.9828, 14.5) -> (11.9828, 14.5)
  line L746 (8.431, 13.5) -> (8.431, 14.5)
  line L747 (9.431, 13.5) -> (8.431, 13.5)
  line L748 (9.431, 14.5) -> (9.431, 13.5)
  line L749 (8.431, 14.5) -> (9.431, 14.5)
  line L750 (5.8793, 13.5) -> (5.8793, 14.5)
  line L751 (6.8793, 13.5) -> (5.8793, 13.5)
  line L752 (6.8793, 14.5) -> (6.8793, 13.5)
  line L753 (5.8793, 14.5) -> (6.8793, 14.5)
  line L754 (3.3276, 13.5) -> (3.3276, 14.5)
  line L755 (4.3276, 13.5) -> (3.3276, 13.5)
  line L756 (4.3276, 14.5) -> (4.3276, 13.5)
  line L757 (3.3276, 14.5) -> (4.3276, 14.5)
  line L758 (0.7759, 13.5) -> (0.7759, 14.5)
  line L759 (1.7759, 13.5) -> (0.7759, 13.5)
  line L760 (1.7759, 14.5) -> (1.7759, 13.5)
  line L761 (0.7759, 14.5) -> (1.7759, 14.5)
  line L762 (-1.7759, 13.5) -> (-1.7759, 14.5)
  line L763 (-0.7759, 13.5) -> (-1.7759, 13.5)
  line L764 (-0.7759, 14.5) -> (-0.7759, 13.5)
  line L765 (-1.7759, 14.5) -> (-0.7759, 14.5)
  line L766 (-4.3276, 13.5) -> (-4.3276, 14.5)
  line L767 (-3.3276, 13.5) -> (-4.3276, 13.5)
  line L768 (-3.3276, 14.5) -> (-3.3276, 13.5)
  line L769 (-4.3276, 14.5) -> (-3.3276, 14.5)
  line L770 (-6.8793, 13.5) -> (-6.8793, 14.5)
  line L771 (-5.8793, 13.5) -> (-6.8793, 13.5)
  line L772 (-5.8793, 14.5) -> (-5.8793, 13.5)
  line L773 (-6.8793, 14.5) -> (-5.8793, 14.5)
  line L774 (-9.431, 13.5) -> (-9.431, 14.5)
  line L775 (-8.431, 13.5) -> (-9.431, 13.5)
  line L776 (-8.431, 14.5) -> (-8.431, 13.5)
  line L777 (-9.431, 14.5) -> (-8.431, 14.5)
  line L778 (-11.9828, 13.5) -> (-11.9828, 14.5)
  line L779 (-10.9828, 13.5) -> (-11.9828, 13.5)
  line L780 (-10.9828, 14.5) -> (-10.9828, 13.5)
  line L781 (-11.9828, 14.5) -> (-10.9828, 14.5)
  line L782 (-14.5345, 13.5) -> (-14.5345, 14.5)
  line L783 (-13.5345, 13.5) -> (-14.5345, 13.5)
  line L784 (-13.5345, 14.5) -> (-13.5345, 13.5)
  line L785 (-14.5345, 14.5) -> (-13.5345, 14.5)
  line L786 (-17.0862, 13.5) -> (-17.0862, 14.5)
  line L787 (-16.0862, 13.5) -> (-17.0862, 13.5)
  line L788 (-16.0862, 14.5) -> (-16.0862, 13.5)
  line L789 (-17.0862, 14.5) -> (-16.0862, 14.5)
  line L790 (-19.6379, 13.5) -> (-19.6379, 14.5)
  line L791 (-18.6379, 13.5) -> (-19.6379, 13.5)
  line L792 (-18.6379, 14.5) -> (-18.6379, 13.5)
  line L793 (-19.6379, 14.5) -> (-18.6379, 14.5)
  line L794 (-22.1897, 13.5) -> (-22.1897, 14.5)
  line L795 (-21.1897, 13.5) -> (-22.1897, 13.5)
  line L796 (-21.1897, 14.5) -> (-21.1897, 13.5)
  line L797 (-22.1897, 14.5) -> (-21.1897, 14.5)
  line L798 (-24.7414, 13.5) -> (-24.7414, 14.5)
  line L799 (-23.7414, 13.5) -> (-24.7414, 13.5)
  line L800 (-23.7414, 14.5) -> (-23.7414, 13.5)
  line L801 (-24.7414, 14.5) -> (-23.7414, 14.5)
  line L802 (-27.2931, 13.5) -> (-27.2931, 14.5)
  line L803 (-26.2931, 13.5) -> (-27.2931, 13.5)
  line L804 (-26.2931, 14.5) -> (-26.2931, 13.5)
  line L805 (-27.2931, 14.5) -> (-26.2931, 14.5)
  line L806 (-29.8448, 13.5) -> (-29.8448, 14.5)
  line L807 (-28.8448, 13.5) -> (-29.8448, 13.5)
  line L808 (-28.8448, 14.5) -> (-28.8448, 13.5)
  line L809 (-29.8448, 14.5) -> (-28.8448, 14.5)
  line L810 (-32.3966, 13.5) -> (-32.3966, 14.5)
  line L811 (-31.3966, 13.5) -> (-32.3966, 13.5)
  line L812 (-31.3966, 14.5) -> (-31.3966, 13.5)
  line L813 (-32.3966, 14.5) -> (-31.3966, 14.5)
  line L814 (-34.9483, 13.5) -> (-34.9483, 14.5)
  line L815 (-33.9483, 13.5) -> (-34.9483, 13.5)
  line L816 (-33.9483, 14.5) -> (-33.9483, 13.5)
  line L817 (-34.9483, 14.5) -> (-33.9483, 14.5)
  line L818 (-37.5, 13.5) -> (-37.5, 14.5)
  line L819 (-36.5, 13.5) -> (-37.5, 13.5)
  line L820 (-36.5, 14.5) -> (-36.5, 13.5)
  line L821 (-37.5, 14.5) -> (-36.5, 14.5)
  line L822 (48, 0) -> (-52, 0) construction
  line L823 (16, -23) -> (16, -24)
  line L824 (28.8448, -8.5) -> (28.8448, -9.5)
  line L825 (13.5, -20.5) -> (13.5, -21.5)
  line L826 (16, -21.5) -> (15, -21.5)
  line L827 (18.5, -21.5) -> (17.5, -21.5)
  line L828 (20, -21.5) -> (20, -20.5)
  line L829 (17.5, -21.5) -> (17.5, -20.5)
  line L830 (-16, -20.5) -> (-15, -20.5)
  line L831 (18.5, -20.5) -> (18.5, -21.5)
  line L832 (-13.5, -24) -> (-13.5, -23)
  line L833 (17.5, -20.5) -> (18.5, -20.5)
  line L834 (31.3966, -4.5) -> (32.3966, -4.5)
  line L835 (31.3966, -7) -> (32.3966, -7)
  line L836 (5.8793, -13.5) -> (5.8793, -14.5)
  line L837 (32.3966, -6) -> (31.3966, -6)
  line L838 (-8.431, -9.5) -> (-8.431, -8.5)
  line L839 (33.9483, -8.5) -> (33.9483, -9.5)
  line L840 (34.9483, -9.5) -> (34.9483, -8.5)
  line L841 (4.5, -21.5) -> (4.5, -20.5)
  line L842 (2, -20.5) -> (3, -20.5)
  line L843 (32.3966, -7) -> (32.3966, -6)
  line L844 (32.3966, -14.5) -> (32.3966, -13.5)
  line L845 (32.3966, -12) -> (32.3966, -11)
  line L846 (33.9483, -9.5) -> (34.9483, -9.5)
  line L847 (0.7759, -12) -> (1.7759, -12)
  line L848 (31.3966, -13.5) -> (31.3966, -14.5)
  line L849 (32.3966, -4.5) -> (32.3966, -3.5)
  line L850 (4.3276, -13.5) -> (3.3276, -13.5)
  line L851 (4.5, -20.5) -> (5.5, -20.5)
  line L852 (3, -23) -> (3, -24)
  line L853 (31.3966, -11) -> (31.3966, -12)
  line L854 (34.9483, -8.5) -> (33.9483, -8.5)
  line L855 (31.3966, -3.5) -> (31.3966, -4.5)
  line L856 (31.3966, -14.5) -> (32.3966, -14.5)
  line L857 (32.3966, -3.5) -> (31.3966, -3.5)
  line L858 (32.3966, -13.5) -> (31.3966, -13.5)
  line L859 (31.3966, -12) -> (32.3966, -12)
  line L860 (3.3276, -12) -> (4.3276, -12)
  line L861 (3, -21.5) -> (2, -21.5)
  line L862 (32.3966, -11) -> (31.3966, -11)
  line L863 (30.5, -23) -> (31.5, -23)
  line L864 (30.5, -24) -> (30.5, -23)
  line L865 (0.7759, -13.5) -> (0.7759, -14.5)
  line L866 (28.8448, -9.5) -> (29.8448, -9.5)
  line L867 (-10, -20.5) -> (-10, -21.5)
  line L868 (4.3276, -14.5) -> (4.3276, -13.5)
  line L869 (29.8448, -8.5) -> (28.8448, -8.5)
  line L870 (29.8448, -9.5) -> (29.8448, -8.5)
  line L871 (31.3966, -6) -> (31.3966, -7)
  line L872 (28.8448, -12) -> (29.8448, -12)
  line L873 (2, -24) -> (2, -23)
  line L874 (28.8448, -11) -> (28.8448, -12)
  line L875 (29.8448, -12) -> (29.8448, -11)
  line L876 (-11, -24) -> (-11, -23)
  line L877 (-10, -24) -> (-11, -24)
  line L878 (-11, -23) -> (-10, -24) construction
  line L879 (1.7759, -14.5) -> (1.7759, -13.5)
  line L880 (28.8448, -4.5) -> (29.8448, -4.5)
  line L881 (29.8448, -3.5) -> (28.8448, -3.5)
  line L882 (28.8448, -3.5) -> (28.8448, -4.5)
  line L883 (3.3276, -13.5) -> (3.3276, -14.5)
  line L884 (29.8448, -11) -> (28.8448, -11)
  line L885 (29.8448, -4.5) -> (29.8448, -3.5)
  line L886 (28.8448, -14.5) -> (29.8448, -14.5)
  line L887 (4.5, -23) -> (5.5, -23)
  line L888 (29, -20.5) -> (29, -21.5)
  line L889 (28, -21.5) -> (28, -20.5)
  line L890 (12.5, -23) -> (13.5, -23)
  line L891 (29, -23) -> (29, -24)
  line L892 (31.5, -20.5) -> (31.5, -21.5)
  line L893 (-16, -24) -> (-16, -23)
  line L894 (-12.5, -20.5) -> (-12.5, -21.5)
  line L895 (-13.5, -20.5) -> (-12.5, -20.5)
  line L896 (20, -24) -> (20, -23)
  line L897 (-12.5, -23) -> (-12.5, -24)
  line L898 (-12.5, -21.5) -> (-13.5, -21.5)
  line L899 (13.5, -23) -> (13.5, -24)
  line L900 (16, -20.5) -> (16, -21.5)
  line L901 (-12.5, -24) -> (-13.5, -24)
  line L902 (18.5, -24) -> (17.5, -24)
  line L903 (1.7759, -9.5) -> (1.7759, -8.5)
  line L904 (1.7759, -11) -> (0.7759, -11)
  line L905 (4.3276, -11) -> (3.3276, -11)
  line L906 (34, -20.5) -> (34, -21.5)
  line L907 (33.9483, -7) -> (34.9483, -7)
  line L908 (35.5, -24) -> (35.5, -23)
  line L909 (34.9483, -7) -> (34.9483, -6)
  line L910 (-5.8793, -6) -> (-6.8793, -6)
  line L911 (-5.8793, -11) -> (-6.8793, -11)
  line L912 (35.5, -23) -> (36.5, -23)
  line L913 (6.8793, -9.5) -> (6.8793, -8.5)
  line L914 (-8.431, -6) -> (-9.431, -6)
  line L915 (0.7759, -8.5) -> (0.7759, -9.5)
  line L916 (-9.431, -6) -> (-9.431, -7)
  line L917 (6.8793, -11) -> (5.8793, -11)
  line L918 (37.5, -9.5) -> (37.5, -8.5)
  line L919 (-9.431, -3.5) -> (-9.431, -4.5)
  line L920 (36.5, -9.5) -> (37.5, -9.5)
  line L921 (-9.431, -7) -> (-8.431, -7)
  line L922 (4.3276, -12) -> (4.3276, -11)
  line L923 (34.9483, -6) -> (33.9483, -6)
  line L924 (6.8793, -12) -> (6.8793, -11)
  line L925 (33.9483, -6) -> (33.9483, -7)
  line L926 (-6.8793, -12) -> (-5.8793, -12)
  line L927 (-6.8793, -3.5) -> (-6.8793, -4.5)
  line L928 (-5.8793, -9.5) -> (-5.8793, -8.5)
  line L929 (36.5, -23) -> (36.5, -24)
  line L930 (5.8793, -9.5) -> (6.8793, -9.5)
  line L931 (37.5, -8.5) -> (36.5, -8.5)
  line L932 (35.5, -23) -> (36.5, -24) construction
  line L933 (5.8793, -11) -> (5.8793, -12)
  line L934 (-8.431, -4.5) -> (-8.431, -3.5)
  line L935 (-10.9828, -12) -> (-10.9828, -11)
  line L936 (36.5, -8.5) -> (36.5, -9.5)
  line L937 (36.5, -20.5) -> (36.5, -21.5)
  line L938 (5.5, -23) -> (4.5, -24) construction
  line L939 (28, -24) -> (28, -23)
  line L940 (-5.8793, -14.5) -> (-5.8793, -13.5)
  line L941 (1.7759, -13.5) -> (0.7759, -13.5)
  line L942 (-5.8793, -13.5) -> (-6.8793, -13.5)
  line L943 (-8.431, -13.5) -> (-9.431, -13.5)
  line L944 (4.5, -24) -> (4.5, -23)
  line L945 (2, -23) -> (3, -23)
  line L946 (28.8448, -6) -> (28.8448, -7)
  line L947 (31.5, -21.5) -> (30.5, -21.5)
  line L948 (-11, -20.5) -> (-10, -20.5)
  line L949 (32.3966, -8.5) -> (31.3966, -8.5)
  line L950 (-9.431, -14.5) -> (-8.431, -14.5)
  line L951 (31.5, -23) -> (31.5, -24)
  line L952 (30.5, -20.5) -> (31.5, -20.5)
  line L953 (5.8793, -14.5) -> (6.8793, -14.5)
  line L954 (28, -20.5) -> (29, -20.5)
  line L955 (31.5, -24) -> (30.5, -24)
  line L956 (2, -21.5) -> (2, -20.5)
  line L957 (0.7759, -14.5) -> (1.7759, -14.5)
  line L958 (31.3966, -8.5) -> (31.3966, -9.5)
  line L959 (-10, -23) -> (-11, -24) construction
  line L960 (-5.5, -24) -> (-5.5, -23)
  line L961 (31.3966, -9.5) -> (32.3966, -9.5)
  line L962 (-5.5, -21.5) -> (-5.5, -20.5)
  line L963 (32.3966, -9.5) -> (32.3966, -8.5)
  line L964 (5.5, -21.5) -> (4.5, -21.5)
  line L965 (29, -21.5) -> (28, -21.5)
  line L966 (-10, -23) -> (-10, -24)
  line L967 (28, -23) -> (29, -23)
  line L968 (-6.8793, -14.5) -> (-5.8793, -14.5)
  line L969 (5.5, -20.5) -> (5.5, -21.5)
  line L970 (5.5, -24) -> (4.5, -24)
  line L971 (-11, -23) -> (-10, -23)
  line L972 (29, -24) -> (28, -24)
  line L973 (6.8793, -13.5) -> (5.8793, -13.5)
  line L974 (3.3276, -7) -> (4.3276, -7)
  line L975 (34, -21.5) -> (33, -21.5)
  line L976 (-2, -23) -> (-2, -24)
  line L977 (0.5, -21.5) -> (-0.5, -21.5)
  line L978 (0.5, -23) -> (0.5, -24)
  line L979 (-2, -24) -> (-3, -24)
  line L980 (-0.5, -24) -> (-0.5, -23)
  line L981 (0.5, -24) -> (-0.5, -24)
  line L982 (34, -24) -> (33, -24)
  line L983 (1.7759, -7) -> (1.7759, -6)
  line L984 (-4.5, -20.5) -> (-4.5, -21.5)
  line L985 (-3, -24) -> (-3, -23)
  line L986 (-0.5, -21.5) -> (-0.5, -20.5)
  line L987 (-3, -23) -> (-2, -23)
  line L988 (-3, -20.5) -> (-2, -20.5)
  line L989 (6.8793, -7) -> (6.8793, -6)
  line L990 (1.7759, -3.5) -> (0.7759, -3.5)
  line L991 (4.3276, -4.5) -> (4.3276, -3.5)
  line L992 (5.8793, -3.5) -> (5.8793, -4.5)
  line L993 (0.7759, -4.5) -> (1.7759, -4.5)
  line L994 (3.3276, -4.5) -> (4.3276, -4.5)
  line L995 (6.8793, -4.5) -> (6.8793, -3.5)
  line L996 (-0.5, -20.5) -> (0.5, -20.5)
  line L997 (-8.431, -7) -> (-8.431, -6)
  line L998 (37.5, -11) -> (36.5, -11)
  line L999 (37.5, -12) -> (37.5, -11)
  line L1000 (5.8793, -4.5) -> (6.8793, -4.5)
  line L1001 (4.3276, -3.5) -> (3.3276, -3.5)
  line L1002 (-10.9828, -7) -> (-10.9828, -6)
  line L1003 (4.3276, -6) -> (3.3276, -6)
  line L1004 (-10.9828, -4.5) -> (-10.9828, -3.5)
  line L1005 (36.5, -11) -> (36.5, -12)
  line L1006 (0.7759, -3.5) -> (0.7759, -4.5)
  line L1007 (33, -21.5) -> (33, -20.5)
  line L1008 (33, -23) -> (34, -23)
  line L1009 (33, -24) -> (33, -23)
  line L1010 (0.5, -20.5) -> (0.5, -21.5)
  line L1011 (6.8793, -6) -> (5.8793, -6)
  line L1012 (3.3276, -3.5) -> (3.3276, -4.5)
  line L1013 (5.8793, -6) -> (5.8793, -7)
  line L1014 (36.5, -12) -> (37.5, -12)
  line L1015 (6.8793, -3.5) -> (5.8793, -3.5)
  line L1016 (0.7759, -7) -> (1.7759, -7)
  line L1017 (4.3276, -7) -> (4.3276, -6)
  line L1018 (5.8793, -7) -> (6.8793, -7)
  line L1019 (-6.8793, -4.5) -> (-5.8793, -4.5)
  line L1020 (33, -20.5) -> (34, -20.5)
  line L1021 (33.9483, -12) -> (34.9483, -12)
  line L1022 (0.7759, -6) -> (0.7759, -7)
  line L1023 (-16, -21.5) -> (-16, -20.5)
  line L1024 (30.5, -21.5) -> (30.5, -20.5)
  line L1025 (-11, -21.5) -> (-11, -20.5)
  line L1026 (-15, -20.5) -> (-15, -21.5)
  line L1027 (16, -24) -> (15, -24)
  line L1028 (15, -21.5) -> (15, -20.5)
  line L1029 (-15, -21.5) -> (-16, -21.5)
  line L1030 (-13.5, -23) -> (-12.5, -23)
  line L1031 (15, -24) -> (15, -23)
  line L1032 (9.431, -3.5) -> (8.431, -3.5)
  line L1033 (8.431, -4.5) -> (9.431, -4.5)
  line L1034 (10.9828, -12) -> (11.9828, -12)
  line L1035 (10.9828, -6) -> (10.9828, -7)
  line L1036 (11.9828, -3.5) -> (10.9828, -3.5)
  line L1037 (-5.5, -23) -> (-4.5, -23)
  line L1038 (10.9828, -8.5) -> (10.9828, -9.5)
  line L1039 (8.431, -11) -> (8.431, -12)
  line L1040 (-4.3276, -7) -> (-3.3276, -7)
  line L1041 (13.5, -21.5) -> (12.5, -21.5)
  line L1042 (-4.5, -24) -> (-5.5, -24)
  line L1043 (-5.5, -20.5) -> (-4.5, -20.5)
  line L1044 (-4.5, -21.5) -> (-5.5, -21.5)
  line L1045 (-0.7759, -7) -> (-0.7759, -6)
  line L1046 (-0.7759, -3.5) -> (-1.7759, -3.5)
  line L1047 (-17.0862, -9.5) -> (-16.0862, -9.5)
  line L1048 (-16, -23) -> (-15, -23)
  line L1049 (11.9828, -4.5) -> (11.9828, -3.5)
  line L1050 (8.431, -12) -> (9.431, -12)
  line L1051 (9.431, -12) -> (9.431, -11)
  line L1052 (-0.7759, -8.5) -> (-1.7759, -8.5)
  line L1053 (-3.3276, -9.5) -> (-3.3276, -8.5)
  line L1054 (11.9828, -9.5) -> (11.9828, -8.5)
  line L1055 (-3.3276, -4.5) -> (-3.3276, -3.5)
  line L1056 (8.431, -6) -> (8.431, -7)
  line L1057 (9.431, -8.5) -> (8.431, -8.5)
  line L1058 (10.9828, -9.5) -> (11.9828, -9.5)
  line L1059 (-0.7759, -6) -> (-1.7759, -6)
  line L1060 (11.9828, -12) -> (11.9828, -11)
  line L1061 (-0.7759, -4.5) -> (-0.7759, -3.5)
  line L1062 (-4.3276, -9.5) -> (-3.3276, -9.5)
  line L1063 (11.9828, -6) -> (10.9828, -6)
  line L1064 (-0.7759, -9.5) -> (-0.7759, -8.5)
  line L1065 (9.431, -6) -> (8.431, -6)
  line L1066 (8.431, -8.5) -> (8.431, -9.5)
  line L1067 (-1.7759, -4.5) -> (-0.7759, -4.5)
  line L1068 (-4.3276, -4.5) -> (-3.3276, -4.5)
  line L1069 (-11.9828, -3.5) -> (-11.9828, -4.5)
  line L1070 (19.6379, -11) -> (18.6379, -11)
  line L1071 (-10.9828, -13.5) -> (-11.9828, -13.5)
  line L1072 (-11.9828, -8.5) -> (-11.9828, -9.5)
  line L1073 (13.5345, -11) -> (13.5345, -12)
  line L1074 (-13.5345, -13.5) -> (-14.5345, -13.5)
  line L1075 (16.0862, -11) -> (16.0862, -12)
  line L1076 (18.6379, -12) -> (19.6379, -12)
  line L1077 (-10.9828, -11) -> (-11.9828, -11)
  line L1078 (-17.0862, -4.5) -> (-16.0862, -4.5)
  line L1079 (-11.9828, -9.5) -> (-10.9828, -9.5)
  line L1080 (13.5345, -13.5) -> (13.5345, -14.5)
  line L1081 (20, -23) -> (21, -23)
  line L1082 (16.0862, -12) -> (17.0862, -12)
  line L1083 (-13.5345, -9.5) -> (-13.5345, -8.5)
  line L1084 (-16.0862, -14.5) -> (-16.0862, -13.5)
  line L1085 (-13.5345, -6) -> (-14.5345, -6)
  line L1086 (-16.0862, -7) -> (-16.0862, -6)
  line L1087 (19.6379, -13.5) -> (18.6379, -13.5)
  line L1088 (-14.5345, -7) -> (-13.5345, -7)
  line L1089 (-14.5345, -11) -> (-14.5345, -12)
  line L1090 (24.7414, -3.5) -> (23.7414, -3.5)
  line L1091 (-36.5, -11) -> (-37.5, -11)
  line L1092 (-28, -21.5) -> (-29, -21.5)
  line L1093 (-28.8448, -13.5) -> (-29.8448, -13.5)
  line L1094 (-37.5, -12) -> (-36.5, -12)